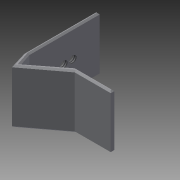
# Autodesk Inventor part: Encoder Mount
Saved by Autodesk Inventor 2015 (Build 190159000, 159)
## iProperties
Created: 2015-04-19
Part Number: Encoder Mount
Material: Generic
Document SubType Name: Modeling
Designer: Kyle
Density: 1 g/cm^3
Appearance: Default
Author: Kyle
Autodesk Inventor part; units mm, degrees
ref_plane "YZ Plane" through (0, 0, 0) normal (1, 0, 0) x (0, 1, 0)
ref_plane "XZ Plane" through (0, 0, 0) normal (0, 1, 0) x (-1, 0, 0)
ref_plane "XY Plane" through (0, 0, 0) normal (0, 0, 1) x (1, 0, 0)
sketch "Sketch1" plane through (0, 0, 0) normal (0, 1, 0) x (-1, 0, 0)
  line L0 (10.2949, -23.8768) -> (10.2949, 26.9232)
  line L1 (10.2949, 26.9232) -> (6.4648, 39.5536)
  line L2 (6.4648, 39.5536) -> (-18.9352, 20.5036)
  line L3 (-18.9352, 20.5036) -> (-44.3352, 20.5036)
  line L4 (-44.3352, 20.5036) -> (-44.3352, 17.9636)
  line L5 (-44.3352, 17.9636) -> (-17.0011, 17.9636)
  line L6 (-17.0011, 17.9636) -> (4.7948, 34.9742)
  line L7 (4.7948, 34.9742) -> (7.7549, 25.8478)
  line L8 (7.7549, 25.8478) -> (7.7549, -23.8768)
  line L9 (7.7549, -23.8768) -> (10.2949, -23.8768)
  point P0 (0, 0)
  dimension "d0" = 19.05
  dimension "d1" = 25.4
  dimension "d2" = 50.8
  dimension "d3" = 70
  dimension "d4" = 70
  dimension "d5" = 2.54
  dimension "d6" = 2.54
  dimension "d7" = 25.4
  constraints: 20 end point, 2 parallel, 2 perpendicular, 2 vertical
  measures "d0" vertical distance of L1.end L2.end
  measures "d1" distance of L2.end L3.end
  measures "d2" distance of L0.start L0.end
  measures "d3" angle of L7 L6
  measures "d4" angle of L1 L2
  measures "d5" distance of L8.end L0.start
  measures "d6" distance of L3.end L4.end
  measures "d7" horizontal distance of L1.end L2.end
extrude "Extrusion1" add sketch "Sketch1" along normal blind 38.1
sketch "Sketch2" plane through (-10.2949, 0, -23.8768) normal (-1, 0, 0) x (0, 0, 1)
  line L0 (19.05, 19.05) -> (25.4, 19.05) construction
  line L1 (25.4, 19.05) -> (25.4, 0) construction
  line L2 (0, 0) -> (50.8, 0) construction
  line L3 (19.05, 19.05) -> (0, 19.05) construction
  line L4 (0, 0) -> (0, 38.1) construction
  point P0 (23.8768, 0)
  dimension "d10" = 19.05
  dimension "d11" = 6.35
  dimension "d12" = 19.05
  constraints: 6 end point, 2 horizontal, 2 midpoint, 1 perpendicular
  measures "d10" distance of L0.end L1.end
  measures "d11" distance of L0.start L0.end
  measures "d12" distance of L0.start L3.end
hole "Hole1" at (-10.2949, 19.05, -4.8268) at (-10.2949, 19.05, 1.5232) direction (1, 0, 0) diameter 4.9784 end through all thread size "1/4-20 UNC" class "2B" standard "ANSI Unified Screw Threads"
chamfer "Chamfer1" distance 1.016 angle 45 20 edges at (-10.2949, 0, 1.5232) (-8.3798, 0, 33.2384) (6.2352, 0, 30.0286) (31.6352, 0, 20.5036) (44.3352, 0, 19.2336) (30.6682, 0, 17.9636) (6.1031, 0, 26.4689) (-6.2749, 0, 30.411) (-7.7549, 0, 0.9855) (-9.0249, 0, -23.8768) (31.6352, 38.1, 20.5036) (44.3352, 38.1, 19.2336) (30.6682, 38.1, 17.9636) (6.2352, 38.1, 30.0286) (6.1031, 38.1, 26.4689) (-6.2749, 38.1, 30.411) (-8.3798, 38.1, 33.2384) (-7.7549, 38.1, 0.9855) (-10.2949, 38.1, 1.5232) (-9.0249, 38.1, -23.8768)
body "Solid1"
